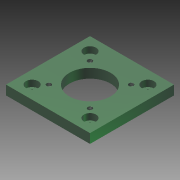
# Autodesk Inventor part: 13_0204_060
Saved by Autodesk Inventor 2012 SP1 (Build 160190100, 190)
## iProperties
Created: 2013-04-29
Part Number: 13_0204_060
Material: Default
Document SubType Name: Modeling
Designer: vogel
Density: 1 g/cm^3
Author: vogel
Autodesk Inventor part; units mm, degrees
ref_plane "YZ Plane" through (0, 0, 0) normal (1, 0, 0) x (0, 1, 0)
ref_plane "XZ Plane" through (0, 0, 0) normal (0, 1, 0) x (-1, 0, 0)
ref_plane "XY Plane" through (0, 0, 0) normal (0, 0, 1) x (1, 0, 0)
sketch "Skizze1" plane through (0, 0, 0) normal (0, 0, 1) x (1, 0, 0)
  line L0 (-22.5, 22.5) -> (22.5, 22.5)
  line L1 (22.5, 22.5) -> (22.5, -22.5)
  line L2 (22.5, -22.5) -> (-22.5, -22.5)
  line L3 (-22.5, -22.5) -> (-22.5, 22.5)
  circle A0 centre (0, 0) radius 11
  line L4 (-31.5, 0) -> (31.5, 0) projected
  line L5 (0, -31.5) -> (0, 31.5) projected
  dimension "d0" = 22
  dimension "d1" = 45
  constraints: 8 end point, 2 parallel, 2 perpendicular, 1 centre point, 1 coincident, 1 horizontal, 2 other
  measures "d0" diameter of A0
  measures "d1" distance of L0.end L1.end
extrude "Extrusion1" add sketch "Skizze1" along normal blind 5 contours L0 L5 A0 L4 L3 | L0 L1 L4 A0 L5 | L4 A0 L5 L2 L3 | L1 L2 L5 A0 L4
sketch "Skizze2" plane through (0, 0, 5) normal (0, 0, 1) x (1, 0, 0)
  line L0 (-11, 11) -> (11, 11)
  line L1 (11, 11) -> (11, -11)
  line L2 (11, -11) -> (-11, -11)
  line L3 (-11, -11) -> (-11, 11)
  line L4 (-31.5, 0) -> (31.5, 0) projected
  line L5 (0, -31.5) -> (0, 31.5) projected
  dimension "d4" = 22
  constraints: 8 end point, 4 coincident, 2 parallel, 2 perpendicular, 1 horizontal, 2 other
  measures "d4" distance of L2.end L0.start
hole "Bohrung1" at (-11, 11, 5) at (11, 11, 5) at (11, -11, 5) at (-11, -11, 5) direction (0, 0, -1) diameter 2.459 end through all thread size "M3x0.5" class "6H" standard "ISO Metric profile"
sketch "Skizze3" plane through (0, 0, 5) normal (0, 0, 1) x (1, 0, 0)
  line L0 (-31.5, 0) -> (31.5, 0) projected
  line L1 (0, -31.5) -> (0, 31.5) projected
  line L2 (-15.5, 15.5) -> (15.5, 15.5)
  line L3 (15.5, 15.5) -> (15.5, -15.5)
  line L4 (15.5, -15.5) -> (-15.5, -15.5)
  line L5 (-15.5, -15.5) -> (-15.5, 15.5)
  dimension "d12" = 31
  constraints: 8 end point, 3 coincident, 2 parallel, 2 perpendicular, 1 horizontal, 2 other
  measures "d12" distance of L2.start L2.end
hole "Bohrung2" at (15.5, -15.5, 5) at (-15.5, 15.5, 5) at (15.5, 15.5, 5) at (-15.5, -15.5, 5) direction (0, 0, -1) diameter 3.4 end through all counterbore diameter 6.5 counterbore depth 3.4
